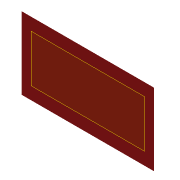
# Autodesk Inventor part: loft version
Saved by Autodesk Inventor 2015 (Build 190159000, 159)
## iProperties
Created: 2015-01-03
Part Number: loft version
Material: Generic
Document SubType Name: Modeling
Designer: Peter
Density: 1 g/cm^3
Appearance: Light Red
Author: Peter
Autodesk Inventor part; units mm, degrees
ref_plane "YZ Plane" through (0, 0, 0) normal (1, 0, 0) x (0, 1, 0)
ref_plane "XZ Plane" through (0, 0, 0) normal (0, 1, 0) x (-1, 0, 0)
sketch "Sketch1" plane through (0, 0, 0) normal (0, 0, 1) x (1, 0, 0)
  line L0 (0, 0) -> (1219.2, 0)
  line L1 (1219.2, 0) -> (1219.2, 508)
  line L2 (1219.2, 508) -> (0, 508)
  line L3 (0, 508) -> (0, 0)
  dimension "d0" = 1219.2
  dimension "d1" = 508
  constraints: 8 end point, 2 parallel, 1 horizontal, 1 perpendicular
  measures "d0" distance of L2.end L1.end
  measures "d1" distance of L1.end L0.end
ref_plane "Work Plane1" through (0, 0, 50.8) normal (0, 0, 1) x (1, 0, 0)
sketch "Sketch2" plane through (0, 0, 50.8) normal (0, 0, 1) x (1, 0, 0)
  line L0 (1219.2, 508) -> (0, 508) projected
  line L1 (0, 508) -> (0, 0) projected
  line L2 (1219.2, 0) -> (1219.2, 508) projected
  line L3 (0, 0) -> (1219.2, 0) projected
  line L4 (-173.736, 681.736) -> (1392.936, 681.736)
  line L5 (1392.936, 681.736) -> (1392.936, -173.736)
  line L6 (1392.936, -173.736) -> (-173.736, -173.736)
  line L7 (-173.736, -173.736) -> (-173.736, 681.736)
  dimension "d3" = 173.736
  constraints: 8 end point, 3 other
  measures "d3" distance between parallel lines of L4 L0
loft "Loft1" add profiles "Sketch1", "Sketch2" contours all / L2 L3 L1 L0 | L4 L5 L6 L7
body "Solid1"
